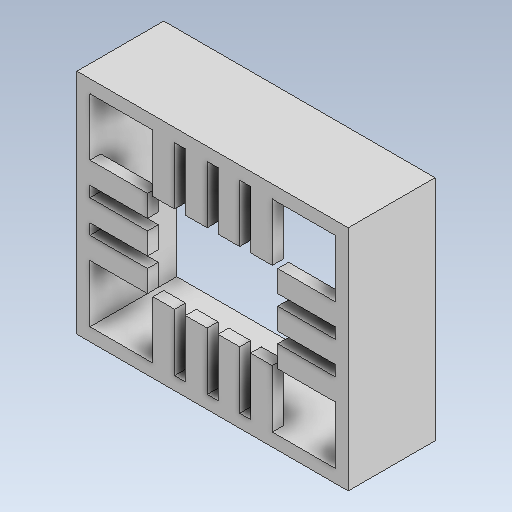
# Autodesk Inventor part: Magazin_2_trichter_4
Saved by Autodesk Inventor 2025.2 (Build 292293000, 293)
## iProperties
Created: 2025-06-21
Part Number: Magazin_2_trichter_4
Material: Generisch
Document SubType Name: Modeling
Designer: maria
Density: 1 g/cm^3
Appearance: Vorgabe
Author: maria
## iProperties of the stored document Magazin_2_trichter_4_3D-Druck.ipt
Created: 2025-06-21
Part Number: Magazin_2_trichter_4_3D-Druck
Material: Generisch
Document SubType Name: Modeling
Designer: maria
Density: 1 g/cm^3
Appearance: Vorgabe
Author: maria
Autodesk Inventor part; units mm, degrees
ref_plane "YZ Plane" through (0, 0, 0) normal (1, 0, 0) x (0, 1, 0)
ref_plane "XZ Plane" through (0, 0, 0) normal (0, 1, 0) x (-1, 0, 0)
ref_plane "XY Plane" through (0, 0, 0) normal (0, 0, 1) x (1, 0, 0)
sketch "Skizze1" plane through (0, 0, 0) normal (0, 1, 0) x (-1, 0, 0)
  line L0 (25.6, 3) -> (-3, 3)
  line L1 (-3, 3) -> (-3, -21.6)
  line L2 (-3, -21.6) -> (25.6, -21.6)
  line L3 (25.6, -21.6) -> (25.6, 3)
  line L4 (22.6, -5.3) -> (17.3, -5.3)
  line L5 (17.3, -5.3) -> (17.3, -7.3)
  line L6 (17.3, -7.3) -> (22.6, -7.3)
  line L7 (22.6, -8.3) -> (17.3, -8.3)
  line L8 (17.3, -8.3) -> (17.3, -10.3)
  line L9 (17.3, -10.3) -> (22.6, -10.3)
  line L10 (22.6, -11.3) -> (17.3, -11.3)
  line L11 (17.3, -11.3) -> (17.3, -13.3)
  line L12 (17.3, -13.3) -> (22.6, -13.3)
  line L13 (0, -5.3) -> (5.3, -5.3)
  line L14 (5.3, -5.3) -> (5.3, -7.3)
  line L15 (5.3, -7.3) -> (0, -7.3)
  line L16 (0, -8.3) -> (5.3, -8.3)
  line L17 (5.3, -10.3) -> (0, -10.3)
  line L18 (0, -11.3) -> (5.3, -11.3)
  line L19 (5.3, -13.3) -> (0, -13.3)
  line L20 (14.8, -18.6) -> (14.8, -13.3)
  line L21 (14.8, -13.3) -> (16.8, -13.3)
  line L22 (16.8, -13.3) -> (16.8, -18.6)
  line L23 (13.8, -13.3) -> (11.8, -13.3)
  line L24 (11.8, -13.3) -> (11.8, -18.6)
  line L25 (13.8, -18.6) -> (13.8, -13.3)
  line L26 (10.8, -13.3) -> (8.8, -13.3)
  line L27 (8.8, -13.3) -> (8.8, -18.6)
  line L28 (10.8, -18.6) -> (10.8, -13.3)
  line L29 (7.8, -13.3) -> (5.8, -13.3)
  line L30 (5.8, -13.3) -> (5.8, -18.6)
  line L31 (7.8, -18.6) -> (7.8, -13.3)
  line L32 (14.8, 0) -> (14.8, -5.3)
  line L33 (16.8, -5.3) -> (16.8, 0)
  line L34 (11.8, -5.3) -> (11.8, 0)
  line L35 (13.8, 0) -> (13.8, -5.3)
  line L36 (8.8, -5.3) -> (8.8, 0)
  line L37 (10.8, 0) -> (10.8, -5.3)
  line L38 (5.8, -5.3) -> (5.8, 0)
  line L39 (7.8, 0) -> (7.8, -5.3)
  line L40 (17.3, -7.3) -> (17.3, -5.3)
  line L41 (17.3, -13.3) -> (17.3, -11.3)
  line L42 (17.3, -10.3) -> (17.3, -8.3)
  line L43 (14.8, -13.3) -> (16.8, -13.3)
  line L44 (11.8, -13.3) -> (13.8, -13.3)
  line L45 (5.3, -5.3) -> (5.3, -7.3)
  line L46 (5.3, -8.3) -> (5.3, -10.3)
  line L47 (5.3, -11.3) -> (5.3, -13.3)
  line L48 (5.8, -13.3) -> (7.8, -13.3)
  line L49 (8.8, -13.3) -> (10.8, -13.3)
  line L50 (7.8, -5.3) -> (5.8, -5.3)
  line L51 (10.8, -5.3) -> (8.8, -5.3)
  line L52 (17.3, -5.3) -> (14.8, -5.3)
  line L53 (13.8, -5.3) -> (11.8, -5.3)
  line L54 (22.6, -10.3) -> (22.6, -11.3)
  line L55 (22.6, -13.3) -> (22.6, -18.6)
  line L56 (22.6, 0) -> (22.6, -5.3)
  line L57 (22.6, -7.3) -> (22.6, -8.3)
  line L58 (22.6, -18.6) -> (16.8, -18.6)
  line L59 (14.8, -18.6) -> (13.8, -18.6)
  line L60 (11.8, -18.6) -> (10.8, -18.6)
  line L61 (8.8, -18.6) -> (7.8, -18.6)
  line L62 (5.8, -18.6) -> (0, -18.6)
  line L63 (0, -18.6) -> (0, -13.3)
  line L64 (0, -5.3) -> (0, 0)
  line L65 (0, -10.3) -> (0, -11.3)
  line L66 (0, -13.3) -> (0, -18.6)
  line L67 (0, -11.3) -> (0, -10.3)
  line L68 (0, -8.3) -> (0, -7.3)
  line L69 (0, 0) -> (0, -5.3)
  line L70 (0, -7.3) -> (0, -8.3)
  line L71 (0, 0) -> (5.8, 0)
  line L72 (7.8, 0) -> (8.8, 0)
  line L73 (10.8, 0) -> (11.8, 0)
  line L74 (13.8, 0) -> (14.8, 0)
  line L75 (16.8, 0) -> (22.6, 0)
  line L76 (23.8, 1.2) -> (-1.2, 1.2)
  line L77 (-1.2, 1.2) -> (-1.2, -19.8)
  line L78 (-1.2, -19.8) -> (23.8, -19.8)
  line L79 (23.8, -19.8) -> (23.8, 1.2)
  dimension "d2" = 12
  dimension "d3" = 8
  dimension "d9" = 24.6
  dimension "d14" = 28.6
  dimension "d21" = 2
  dimension "d22" = 2
  dimension "d23" = 2
  dimension "d24" = 1
  dimension "d25" = 1
  dimension "d26" = 2
  dimension "d27" = 2
  dimension "d28" = 2
  dimension "d29" = 2
  dimension "d30" = 1
  dimension "d31" = 1
  dimension "d32" = 1
  dimension "d33" = 0.5
  dimension "d34" = 0.5
  dimension "d43" = 21
  dimension "d44" = 25
  dimension "d50" = 3
  dimension "d51" = 1.8
  dimension "d52" = 1.8
  dimension "d54" = 1.8
  constraints: 160 end point, 77 parallel, 40 perpendicular, 17 horizontal
  measures "d2" distance of L19.start L11.end
  measures "d3" distance of L11.end L40.end
  measures "d9" distance of L0.end L1.end
  measures "d14" distance between parallel lines of L1 L3
  measures "d21" distance of L11.end L10.end
  measures "d22" distance of L7.end L8.end
  measures "d23" distance of L4.end L5.end
  measures "d24" distance between parallel lines of L10 L9
  measures "d25" distance between parallel lines of L7 L6
  measures "d26" distance between parallel lines of L22 L20
  measures "d27" distance between parallel lines of L24 L25
  measures "d28" distance between parallel lines of L27 L28
  measures "d29" distance between parallel lines of L30 L31
  measures "d30" distance between parallel lines of L27 L31
  measures "d31" distance between parallel lines of L24 L28
  measures "d32" distance between parallel lines of L20 L25
  measures "d33" distance from line of L11.end L22
  measures "d34" distance from line of L30 L19.start
  measures "d43" distance of L76.end L77.end
  measures "d44" distance of L77.end L78.end
  measures "d50" distance between parallel lines of L3 L56
  measures "d51" distance between parallel lines of L0 L76
  measures "d52" distance between parallel lines of L2 L78
  measures "d54" distance between parallel lines of L77 L1
extrude "Extrusion1" add sketch "Skizze1" along normal blind 1 contours L79 L78 L77 L76
sketch "Skizze3" plane through (0, 1, 0) normal (0, 1, 0) x (1, 0, 0)
  line L0 (-25.6, -3) -> (3, -3) projected
  line L1 (3, -3) -> (3, 21.6) projected
  line L2 (-25.6, -3) -> (3, -3)
  line L3 (3, -3) -> (3, 21.6)
  line L4 (3, 21.6) -> (-25.6, 21.6)
  line L5 (-25.6, 21.6) -> (-25.6, -3)
  line L6 (-24.1, -1.5) -> (1.5, -1.5)
  line L7 (1.5, -1.5) -> (1.5, 20.1)
  line L8 (1.5, 20.1) -> (-24.1, 20.1)
  line L9 (-24.1, 20.1) -> (-24.1, -1.5)
  line L10 (1.2, 19.8) -> (-23.8, 19.8) projected
  line L11 (1.2, -1.2) -> (1.2, 19.8) projected
  line L12 (-23.8, 19.8) -> (1.2, 19.8)
  line L13 (1.2, 19.8) -> (1.2, -1.2)
  line L14 (1.2, -1.2) -> (-23.8, -1.2)
  line L15 (-23.8, -1.2) -> (-23.8, 19.8)
  line L16 (-22.6, 13.3) -> (-22.6, 18.6) projected
  line L17 (-22.6, 18.6) -> (0, 18.6)
  line L18 (0, 18.6) -> (0, 0)
  line L19 (0, 0) -> (-22.6, 0)
  line L20 (-22.6, 0) -> (-22.6, 18.6)
  dimension "d37" = 1.5
  dimension "d38" = 1.5
  dimension "d39" = 1.5
  dimension "d40" = 1.5
  constraints: 32 end point, 8 parallel, 4 horizontal, 4 perpendicular
  measures "d37" distance between parallel lines of L4 L8
  measures "d38" distance between parallel lines of L5 L9
  measures "d39" distance between parallel lines of L0 L6
  measures "d40" distance between parallel lines of L1 L7
extrude "Extrusion2" add sketch "Skizze3" along normal blind 7 contours L11 L14 L15 L10
